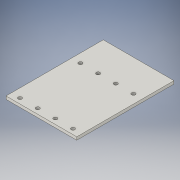
# Autodesk Inventor part: Z Adapter
Saved by Autodesk Inventor 2018.2 (Build 222227000, 227)
## iProperties
Created: 2018-01-21
Part Number: Z Adapter
Material: Steel
Document SubType Name: Modeling
Designer: torba
Density: 7.85 g/cm^3
Appearance: Steel
Author: torba
Autodesk Inventor part; units mm, degrees
ref_plane "YZ Plane" through (0, 0, 0) normal (1, 0, 0) x (0, 1, 0)
ref_plane "XZ Plane" through (0, 0, 0) normal (0, 1, 0) x (-1, 0, 0)
ref_plane "XY Plane" through (0, 0, 0) normal (0, 0, 1) x (1, 0, 0)
sketch "Sketch1" plane through (0, 0, 0) normal (0, 1, 0) x (-1, 0, 0)
  circle A0 centre (165.1, 11.1125) radius 3.9687
  circle A1 centre (127, 11.1125) radius 3.9687
  circle A2 centre (88.9, 11.1125) radius 3.9687
  circle A3 centre (50.8, 11.1125) radius 3.9687
  circle A4 centre (50.8, 141.2875) radius 3.9687
  circle A5 centre (88.9, 141.2875) radius 3.9687
  circle A6 centre (127, 141.2875) radius 3.9687
  circle A7 centre (165.1, 141.2875) radius 3.9687
  spline S0 degree 3 poles (123.0312, 11.1125) (123.0312, 10.8098) (123.0634, 10.5466) (123.1694, 10.0431) (123.2446, 9.8041) (123.5396, 9.1042) (123.8315, 8.6683) (124.5166, 7.9833) (124.9379, 7.6805) (125.6663, 7.3652) (125.925, 7.2825) (126.4569, 7.1717) (126.7301, 7.1437) (127.2699, 7.1437) (127.5431, 7.1717) (128.075, 7.2825) (128.3337, 7.3652) (129.0621, 7.6805) (129.4834, 7.9833) (130.1685, 8.6683) (130.4604, 9.1042) (130.7554, 9.8041) (130.8306, 10.0431) (130.9366, 10.5466) (130.9687, 10.8098) (130.9687, 11.4152) (130.9366, 11.6784) (130.8306, 12.1819) (130.7554, 12.4209) (130.4604, 13.1208) (130.1685, 13.5567) (129.4834, 14.2417) (129.0621, 14.5445) (128.3337, 14.8598) (128.075, 14.9425) (127.5431, 15.0533) (127.2699, 15.0812) (126.7301, 15.0812) (126.4569, 15.0533) (125.925, 14.9425) (125.6663, 14.8598) (124.9379, 14.5445) (124.5166, 14.2417) (123.8315, 13.5567) (123.5396, 13.1208) (123.2446, 12.4209) (123.1694, 12.1819) (123.0634, 11.6784) (123.0312, 11.4152) (123.0312, 11.1125) knots -2.748717 -2.748717 -2.748717 -2.748717 -2.657901 -2.657901 -2.567085 -2.567085 -2.385454 -2.385454 -2.223496 -2.223496 -2.142517 -2.142517 -2.061538 -2.061538 -1.980559 -1.980559 -1.89958 -1.89958 -1.737622 -1.737622 -1.55599 -1.55599 -1.465174 -1.465174 -1.374359 -1.374359 -1.283543 -1.283543 -1.192727 -1.192727 -1.011095 -1.011095 -0.849137 -0.849137 -0.768158 -0.768158 -0.687179 -0.687179 -0.6062 -0.6062 -0.525221 -0.525221 -0.363263 -0.363263 -0.181632 -0.181632 -0.090816 -0.090816 0 0 0 0
  line L0 (0, 0) -> (215.9, 0)
  line L1 (215.9, 0) -> (215.9, 152.4)
  line L2 (215.9, 152.4) -> (0, 152.4)
  line L3 (0, 152.4) -> (0, 0)
  line L4 (215.9, 0) -> (0, 0)
  line L5 (0, 0) -> (0, -6.35)
  line L6 (0, -6.35) -> (215.9, -6.35)
  line L7 (215.9, -6.35) -> (215.9, 0)
  line L8 (215.9, -6.35) -> (0, -6.35)
  line L9 (0, -6.35) -> (0, -57.15)
  line L10 (0, -57.15) -> (215.9, -57.15)
  line L11 (215.9, -57.15) -> (215.9, -6.35)
  dimension "d0" = 215.9
  dimension "d1" = 152.4
  dimension "d2" = 6.35
  dimension "d3" = 50.8
  dimension "d4" = 7.9375
  dimension "d8" = 215.9
  dimension "d12" = 50.8
  dimension "d13" = 11.1125
  dimension "d14" = 50.8
  dimension "d15" = 141.2875
  dimension "d16" = 88.9
  dimension "d17" = 11.1125
  dimension "d18" = 88.9
  dimension "d19" = 141.2875
  dimension "d20" = 92.8688
  dimension "d21" = 141.2875
  dimension "d22" = 127
  dimension "d23" = 11.1125
  dimension "d24" = 127
  dimension "d25" = 141.2875
  dimension "d26" = 165.1
  dimension "d27" = 11.1125
  dimension "d28" = 165.1
  dimension "d29" = 141.2875
  constraints: 24 end point, 7 centre point, 6 equal radius, 6 parallel, 3 horizontal, 3 perpendicular, 1 horizontal alignment, 1 point on line, 3 other
  measures "d0" distance of L2.end L1.end
  measures "d1" distance of L1.end L0.end
  measures "d2" distance of L5.end L4.end
  measures "d3" distance of L9.end L8.end
  measures "d4" diameter of A7
  measures "d8" distance between parallel lines of L11 L9
  measures "d12" distance from line of A7.centre L11
  measures "d13" distance from line of A7.centre L2
  measures "d14" distance from line of A0.centre L11
  measures "d15" distance from line of A0.centre L2
  measures "d16" distance from line of A6.centre L11
  measures "d17" distance from line of A6.centre L2
  measures "d18" distance from line of point (127, 11.112) L11
  measures "d19" distance from line of point (127, 11.112) L2
  measures "d20" distance from line of point (123.031, 11.112) L11
  measures "d21" distance from line of point (123.031, 11.112) L2
  measures "d22" distance from line of A5.centre L11
  measures "d23" distance from line of A5.centre L2
  measures "d24" distance from line of A2.centre L11
  measures "d25" distance from line of A2.centre L2
  measures "d26" distance from line of A4.centre L11
  measures "d27" distance from line of A4.centre L2
  measures "d28" distance from line of A3.centre L11
  measures "d29" distance from line of A3.centre L2
extrude "Extrusion1" add sketch "Sketch1" along normal blind 6.35
sketch "Sketch2" plane through (0, 0, 0) normal (0, -1, 0) x (1, 0, 0)
  circle A0 centre (-165.1, 141.2875) radius 3.9687 projected
  circle A1 centre (-50.8, 11.1125) radius 3.9687 projected
  circle A2 centre (-88.9, 11.1125) radius 3.9687 projected
  circle A3 centre (-50.8, 141.2875) radius 3.9687 projected
  circle A4 centre (-88.9, 141.2875) radius 3.9687 projected
  circle A5 centre (-165.1, 11.1125) radius 3.9687 projected
  circle A6 centre (-127, 141.2875) radius 3.9687 projected
  line L0 (-215.9, -57.15) -> (-215.9, 152.4) projected
  line L1 (0, -57.15) -> (-215.9, -57.15) projected
  line L2 (0, 152.4) -> (0, -57.15) projected
  line L3 (-215.9, 152.4) -> (0, 152.4) projected
  line L4 (0, 152.4) -> (0, -57.15) projected
  line L5 (0, -57.15) -> (-215.9, -57.15) projected
  line L6 (0, 152.4) -> (-31.75, 152.4)
  line L7 (-31.75, 152.4) -> (-31.75, -57.15)
  line L8 (-31.75, -57.15) -> (0, -57.15)
  line L9 (0, -57.15) -> (0, 152.4)
  line L10 (-215.9, 152.4) -> (-184.15, 152.4)
  line L11 (-184.15, 152.4) -> (-184.15, -57.15)
  line L12 (-184.15, -57.15) -> (-215.9, -57.15)
  line L13 (-215.9, -57.15) -> (-215.9, 152.4)
  point P0 (0, 0)
  dimension "d34" = 31.75
  dimension "d35" = 31.75
  constraints: 16 end point, 4 parallel, 2 horizontal, 2 perpendicular, 2 point on line, 1 other
  measures "d34" distance of L8.end L7.end
  measures "d35" distance of L11.end L12.end
extrude "Extrusion2" cut sketch "Sketch2" against normal blind 6.35 contours L0 L3 L11 L1 | L7 L3 L2 L1
body "Solid1"
